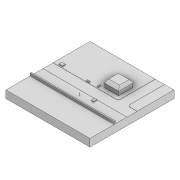
# Autodesk Inventor part: scene1
Saved by Autodesk Inventor 2021 (Build 250183000, 183)
## iProperties
Created: 2022-03-08
Part Number: scene1
Material: Generic
Document SubType Name: Modeling
Designer: Derm
Density: 1 g/cm^3
Appearance: Default
Author: Derm
Autodesk Inventor part; units mm, degrees
ref_plane "YZ Plane" through (0, 0, 0) normal (1, 0, 0) x (0, 1, 0)
ref_plane "XZ Plane" through (0, 0, 0) normal (0, 1, 0) x (-1, 0, 0)
sketch "Sketch1" plane through (0, 0, 0) normal (0, 1, 0) x (-1, 0, 0)
  line L0 (50000, 50000) -> (-50000, 50000)
  line L1 (-50000, 50000) -> (-50000, -50000)
  line L2 (-50000, -50000) -> (50000, -50000)
  line L3 (50000, -50000) -> (50000, 50000)
  line L4 (50000, 50000) -> (-50000, -50000) construction
  line L5 (-50000, 50000) -> (50000, -50000) construction
  point P0 (0, 0)
  dimension "d0" = 100000
  dimension "d1" = 100000
  constraints: 12 end point, 2 midpoint, 2 parallel, 1 horizontal, 1 perpendicular
  measures "d0" distance of L1.end L2.end
  measures "d1" distance of L0.end L1.end
extrude "Extrusion1" add sketch "Sketch1" against normal blind 3000
sketch "Sketch2" plane through (0, 0, 0) normal (0, 1, 0) x (1, 0, 0)
  line L0 (50000, -50000) -> (50000, 50000) projected
  line L1 (50000, 50000) -> (-50000, 50000) projected
  line L2 (-50000, 50000) -> (-50000, -50000) projected
  line L3 (-50000, -50000) -> (50000, -50000) projected
  line L4 (50000, 50000) -> (50000, -50000) projected
  line L5 (-50000, -6000) -> (50000, -6000)
  line L6 (50000, -6000) -> (50000, 6000)
  line L7 (-50000, 6000) -> (-50000, -6000)
  line L8 (-50000, -6000) -> (50000, 6000) construction
  line L9 (50000, -6000) -> (-50000, 6000) construction
  line L10 (-50000, 50000) -> (50000, 50000) projected
  line L11 (38735.1966, 9000) -> (38735.1966, 50000)
  line L12 (38735.1966, 50000) -> (27735.1966, 50000)
  line L13 (27735.1966, 50000) -> (27735.1966, 9000)
  line L14 (50000, 6000) -> (41735.1966, 6000)
  line L15 (24735.1966, 6000) -> (-50000, 6000)
  arc A0 (24735.1966, 6000) -> (27735.1966, 9000) centre (24735.1966, 9000) ccw
  arc A1 (38735.1966, 9000) -> (41735.1966, 6000) centre (41735.1966, 9000) ccw
  point P0 (0, 0)
  dimension "d5" = 11000
  dimension "d6" = 3000
  constraints: 20 end point, 4 parallel, 4 point on circle, 4 tangent, 2 centre point, 2 midpoint, 2 point on line, 1 equal radius, 1 horizontal, 1 perpendicular
  measures "d5" distance between parallel lines of L11 L13
  measures "d6" radius of A0
extrude "Extrusion2" cut sketch "Sketch2" against normal blind 100 contours L5 L2 L15 A0 L13 L1 L11 A1 L14 L0
sketch "Sketch3" plane through (0, 0, 0) normal (0, 1, 0) x (1, 0, 0)
  line L0 (50000, 50000) -> (50000, -50000) projected
  line L1 (50000, -50000) -> (-50000, -50000) projected
  line L2 (-50000, -50000) -> (-50000, 50000) projected
  line L3 (-50000, 50000) -> (50000, 50000) projected
  line L4 (-50000, 6000) -> (24735.1966, 6000) projected
  arc A0 (24735.1966, 6000) -> (27735.1966, 9000) centre (24735.1966, 9000) ccw projected
  line L5 (27735.1966, 9000) -> (27735.1966, 50000) projected
  line L6 (27735.1966, 50000) -> (-50000, 50000) projected
  line L7 (-50000, 50000) -> (-50000, 6000) projected
  line L8 (23068.1077, 10876.2035) -> (6908.7226, 10876.2035)
  line L9 (6908.7226, 10876.2035) -> (6908.7226, 28000)
  line L10 (6908.7226, 28000) -> (23068.1077, 28000)
  line L11 (23068.1077, 28000) -> (23068.1077, 10876.2035)
  line L12 (23068.1077, 10876.2035) -> (6908.7226, 28000) construction
  line L13 (6908.7226, 10876.2035) -> (23068.1077, 28000) construction
  point P0 (0, 0)
  point P1 (14988.4151, 19438.1018)
  constraints: 12 end point, 2 midpoint, 2 parallel, 1 horizontal, 1 perpendicular
extrude "Extrusion3" add sketch "Sketch3" along normal blind 5000 contours L8 L9 L10 L11
sketch "Sketch4" plane through (23068.1077, 0, -28000) normal (0, 0, -1) x (-1, 0, 0)
  line L0 (16159.3851, 0) -> (0, 0) projected
  line L1 (16159.3851, 0) -> (16159.3851, 5000) projected
  line L2 (0, 5000) -> (16159.3851, 5000) projected
  line L3 (0, 0) -> (0, 5000) projected
  line L4 (0, 5000) -> (16159.3851, 5000) projected
  line L5 (0, 5000) -> (-502.206, 5000)
  line L6 (-502.206, 5000) -> (1674.3292, 8799.2208)
  line L7 (1674.3292, 8799.2208) -> (8079.6925, 8799.2208)
  line L8 (8079.6925, 5000) -> (8079.6925, 8799.2208)
  line L9 (16159.3851, 5000) -> (16661.5911, 5000)
  line L10 (16661.5911, 5000) -> (14485.0559, 8799.2208)
  line L11 (14485.0559, 8799.2208) -> (8079.6925, 8799.2208)
  point P0 (23068.1077, 0)
  constraints: 14 end point, 2 symmetric about line, 1 horizontal, 1 midpoint, 1 parallel, 1 perpendicular
extrude "Extrusion4" add sketch "Sketch4" against normal up to surface (17123.7965 mm away) contours L2 L8 L11 L10 L9 | L5 L6 L7 L8 L2
sketch "Sketch5" plane through (6908.7226, 0, -10876.2035) normal (0, 0, 1) x (1, 0, 0)
  line L0 (16159.3851, 0) -> (0, 0) projected
  line L1 (16159.3851, 0) -> (16159.3851, 5000) projected
  line L2 (16661.5911, 5000) -> (16159.3851, 5000) projected
  line L3 (14485.0559, 8799.2208) -> (16661.5911, 5000) projected
  line L4 (1674.3292, 8799.2208) -> (14485.0559, 8799.2208) projected
  line L5 (-502.206, 5000) -> (1674.3292, 8799.2208) projected
  line L6 (0, 5000) -> (-502.206, 5000) projected
  line L7 (0, 0) -> (0, 5000) projected
  line L8 (0, 5000) -> (-502.206, 5000) projected
  line L9 (16661.5911, 5000) -> (16159.3851, 5000) projected
  line L10 (0, 5000) -> (16159.3851, 5000)
  point P0 (-6908.7226, 0)
  constraints: 2 end point, 1 collinear
extrude "Extrusion5" add sketch "Sketch5" along normal blind 600 contours L10 L6 L5 L4 L3 L2
ref_plane "Work Plane1" through (23068.1077, 0, -19438.1018) normal (0, 0, -1) x (-1, 0, 0)
mirror "Mirror1" about plane through (23068.1077, 0, -19438.1018) normal (0, 0, -1) of "Extrusion5"
chamfer "Chamfer1" distance 50 angle 45 7 edges at (-12632.4017, 0, -6000) (26856.517, 0, -6878.6797) (27735.1966, 0, -29500) (0, 0, 6000) (38735.1966, 0, -29500) (39613.8763, 0, -6878.6797) (45867.5983, 0, -6000)
chamfer "Chamfer2" distance 3500 angle 45 2 edges at (14988.4151, 8799.2208, -10276.2035) (14988.4151, 8799.2208, -28600)
sketch "Sketch6" plane through (0, 0, 0) normal (0, 1, 0) x (1, 0, 0)
  line L0 (-50000, -6050) -> (50000, -6050) projected
  line L1 (-50000, -6050) -> (-50000, -50000) projected
  line L2 (-50000, -50000) -> (50000, -50000) projected
  line L3 (50000, -50000) -> (50000, -6050) projected
  circle A0 centre (0, -12422.6788) radius 250
  point P0 (0, 0)
  dimension "d21" = 500
  dimension "d23" = 37577.3212
  constraints: 1 centre point
  measures "d21" diameter of A0
  measures "d23" distance from line of L2 A0.centre
extrude "Extrusion6" add sketch "Sketch6" along normal blind 3000 contours A0
pattern_linear "Rectangular Pattern1" [suppressed]
sketch "Sketch7" plane through (0, 0, 0) normal (0, 1, 0) x (1, 0, 0)
  circle A0 centre (0, -12422.6788) radius 250 projected
  line L0 (-50000, -6050) -> (50000, -6050) projected
  line L1 (-50000, -6050) -> (-50000, -50000) projected
  line L2 (-50000, -50000) -> (50000, -50000) projected
  line L3 (50000, -50000) -> (50000, -6050) projected
  line L4 (-50000, -6050) -> (-50000, -50000) projected
  line L5 (50000, 50000) -> (50000, -50000) projected
  line L6 (-50000, -21203.5733) -> (50000, -21203.5733)
  line L7 (50000, -21203.5733) -> (50000, -19751.467)
  line L8 (50000, -19751.467) -> (-50000, -19751.467)
  line L9 (-50000, -19751.467) -> (-50000, -21203.5733)
  point P0 (0, 0)
  point P1 (-50000, -19751.467)
  point P2 (50000, -21203.5733)
  constraints: 8 end point, 2 parallel, 2 point on line, 1 horizontal, 1 perpendicular
extrude "Extrusion7" add sketch "Sketch7" along normal blind 3000 contours L8 L3 L6 L1
sketch "Sketch8" plane through (0, 0, 0) normal (0, 1, 0) x (1, 0, 0)
  line L0 (27685.1966, 50000) -> (27685.1966, 9000) projected
  line L1 (27685.1966, 50000) -> (-50000, 50000) projected
  line L2 (-50000, 50000) -> (-50000, 6050) projected
  line L3 (24735.1966, 6050) -> (-50000, 6050) projected
  arc A0 (24735.1966, 6050) -> (27685.1966, 9000) centre (24735.1966, 9000) ccw projected
  line L4 (23068.1077, 28000) -> (23068.1077, 10876.2035) projected
  line L5 (23068.1077, 10876.2035) -> (6908.7226, 10876.2035) projected
  line L6 (6908.7226, 10876.2035) -> (6908.7226, 28000) projected
  line L7 (6908.7226, 28000) -> (23068.1077, 28000) projected
  line L8 (-50000, -19751.467) -> (50000, -19751.467) projected
  line L9 (50000, -19751.467) -> (50000, -6050) projected
  line L10 (-50000, -6050) -> (50000, -6050) projected
  line L11 (-50000, -6050) -> (-50000, -19751.467) projected
  circle A1 centre (0, -12422.6788) radius 250 projected
  line L12 (-7755.2468, 8091.4966) -> (-10970.7872, 8091.4966)
  line L13 (-10970.7872, 8091.4966) -> (-10970.7872, 6734.1239)
  line L14 (-10970.7872, 6734.1239) -> (-7755.2468, 6734.1239)
  line L15 (-7755.2468, 6734.1239) -> (-7755.2468, 8091.4966)
  line L16 (-3927.8334, -1038.8233) -> (-1060.9343, -1038.8233)
  line L17 (-1060.9343, -1038.8233) -> (-1060.9343, -3437.3677)
  line L18 (-1060.9343, -3437.3677) -> (-3927.8334, -3437.3677)
  line L19 (-3927.8334, -3437.3677) -> (-3927.8334, -1038.8233)
  line L20 (-22605.2556, -1038.8233) -> (-21044.0729, -1038.8233)
  line L21 (-21044.0729, -1038.8233) -> (-21044.0729, -5069.5133)
  line L22 (-21044.0729, -5069.5133) -> (-22605.2556, -5069.5133)
  line L23 (-22605.2556, -5069.5133) -> (-22605.2556, -1038.8233)
  line L24 (1181.4921, 10442.9662) -> (2529.7862, 10442.9662)
  line L25 (2529.7862, 10442.9662) -> (2529.7862, 7412.8102)
  line L26 (2529.7862, 7412.8102) -> (1181.4921, 7412.8102)
  line L27 (1181.4921, 7412.8102) -> (1181.4921, 10442.9662)
  line L28 (-44526.7154, 10876.2035) -> (-40062.1541, 10876.2035)
  line L29 (-40062.1541, 10876.2035) -> (-40062.1541, 7412.8102)
  line L30 (-40062.1541, 7412.8102) -> (-44526.7154, 7412.8102)
  line L31 (-44526.7154, 7412.8102) -> (-44526.7154, 10876.2035)
  line L32 (12401.1238, -6673.6776) -> (15000, -6673.6776)
  line L33 (15000, -6673.6776) -> (15000, -10794.2169)
  line L34 (15000, -10794.2169) -> (12401.1238, -10794.2169)
  line L35 (12401.1238, -10794.2169) -> (12401.1238, -6673.6776)
  point P0 (0, 0)
  constraints: 48 end point, 12 parallel, 6 horizontal, 6 perpendicular, 2 point on line
extrude "Extrusion8" add sketch "Sketch8" along normal blind 1000 contours L15 L14 L13 L12 | L24 L25 L26 L27 | L28 L29 L30 L31 | L32 L33 L34 L35
sketch "Sketch9" plane through (0, 0, 0) normal (0, 1, 0) x (1, 0, 0)
  circle A0 centre (-7079.3551, -7895.0186) radius 1405.5966
  circle A1 centre (-3459.7598, 8393.1608) radius 825.3947
  circle A2 centre (15217.3522, 7567.766) radius 874.7148
  circle A3 centre (6747.4991, -9300.6152) radius 1543.0453
  point P0 (0, 0)
  constraints: 4 centre point
extrude "Extrusion9" [suppressed]
sketch "Sketch10" plane through (0, -3000, 0) normal (0, -1, 0) x (1, 0, 0)
  line L0 (50000, -50000) -> (50000, 50000) projected
  line L1 (50000, 50000) -> (-50000, 50000) projected
  line L2 (-50000, 50000) -> (-50000, -50000) projected
  line L3 (-50000, -50000) -> (50000, -50000) projected
  point P0 (0, 0)
extrude "Extrusion10" add sketch "Sketch10" along normal blind 5999.2209
body "Solid1"
